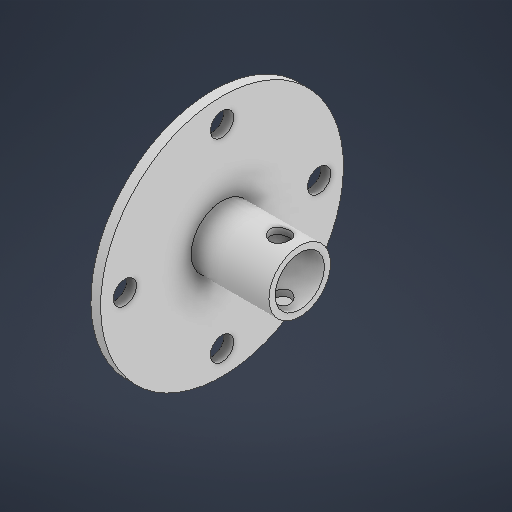
# Autodesk Inventor part: Hub
Saved by Autodesk Inventor 2026.1 (Build 301233000, 233)
## iProperties
Created: 2026-06-12
Part Number: Hub
Material: Generic
Document SubType Name: Modeling
Designer: share
Density: 1 g/cm^3
Appearance: Default
Author: share
Autodesk Inventor part; units mm, degrees
ref_plane "YZ Plane" through (0, 0, 0) normal (1, 0, 0) x (0, 1, 0)
ref_plane "XY Plane" through (0, 0, 0) normal (0, 0, 1) x (1, 0, 0)
sketch "Sketch1" plane through (0, 0, 0) normal (1, 0, 0) x (0, 1, 0)
  circle A0 centre (0, 0) radius 62.5
  dimension "d2" = 125
  constraints: 1 centre point, 1 coincident
  measures "d2" diameter of A0
extrude "Hub Face" add sketch "Sketch1" along normal blind 5
sketch "Sketch2" plane through (5, 0, 0) normal (1, 0, 0) x (0, 0, -1)
  circle A0 centre (0, 0) radius 50 construction
  circle A1 centre (0, 50) radius 6
  line L0 (0, 50) -> (0, 0) construction
  dimension "d4" = 100
  dimension "d3" = 12
  constraints: 2 end point, 1 centre point, 1 coincident, 1 vertical, 1 vertical alignment, 2 other
  measures "d3" diameter of A1
extrude "Lug Bolt Hole" cut sketch "Sketch2" against normal up to surface (5 mm away)
pattern_circular "Lug Bolt Hole Pattern" count 4 over 360 about axis through (-10, 0, 0) along (1, 0, 0) of "Lug Bolt Hole"
sketch "Sketch3" plane through (5, 0, 0) normal (1, 0, 0) x (0, 0, -1)
  circle A0 centre (0, 0) radius 15.875
  circle A1 centre (0, 0) radius 12.7
  dimension "d10" = 31.75
  dimension "d19" = 25.4
  constraints: 2 centre point, 2 coincident
  measures "d10" diameter of A0
  measures "d19" diameter of A1
extrude "Hub Shaft" add sketch "Sketch3" along normal blind 40
ref_plane "Lock Pin Hole Plane" through (0, 15.875, 0) normal (0, 1, 0) x (-1, 0, 0)
sketch "Sketch4" plane through (0, 15.875, 0) normal (0, 1, 0) x (-1, 0, 0)
  line L0 (-45, 15.875) -> (-45, -15.875) projected
  circle A0 centre (-35, 0) radius 5
  point P0 (0, 0)
  dimension "d21" = 10
  dimension "d22" = 10
  constraints: 1 centre point
  measures "d21" diameter of A0
  measures "d22" distance from line of L0 A0.centre
extrude "Extrusion4" cut sketch "Sketch4" against normal through all
equation "\"d2\" = Hub_Diameter"
equation "\"d0\" = Hub_Thickness"
equation "\"d4\" = Lug_Bolt_Pattern_Diameter"
equation "\"d3\" = Lug_Bolt_Hole_Diameter"
equation "\"d10\" = Hub_Shaft_Outer_Diameter"
equation "\"d19\" = Hub_Shaft_Inner_Diameter"
equation "\"d17\" = Hub_Shaft_Length"
equation "\"d21\" = Lock_Pin_Diameter"
equation "\"d22\" = Lock_Pin_Edge_Distance"
equation "\"Hub_Thickness\" = 5"
equation "\"Hub_Diameter\" = 125"
equation "\"Lug_Bolt_Hole_Diameter\" = 12"
equation "\"Hub_Shaft_Diameter\" = 1"
equation "\"Hub_Shaft_Wall_Thickness\" = 1"
equation "\"Hub_Shaft_Length\" = 40"
equation "\"Hub_Shaft_Inner_Diameter\" = 25.4"
equation "\"Hub_Shaft_Outer_Diameter\" = 31.75"
equation "\"d20\" = 0.5 * Hub_Shaft_Outer_Diameter"
equation "\"Lock_Pin_Diameter\" = 10"
equation "\"Lock_Pin_Edge_Distance\" = 10"
equation "\"Lug_Bolt_Pattern_Diameter\" = 100"
body "Solid1"
